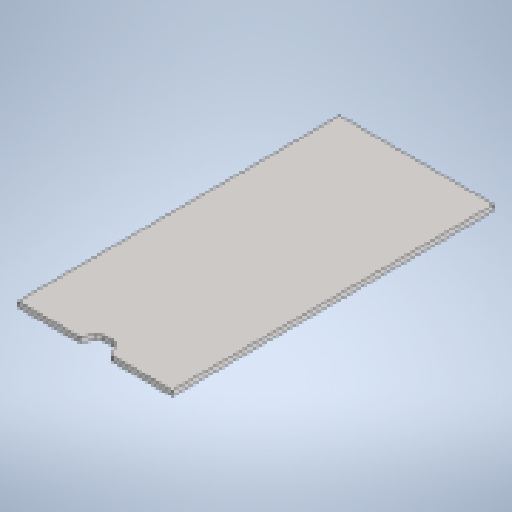
# Autodesk Inventor part: поперечная грань тела
Saved by Autodesk Inventor 2023.1 (Build 271208000, 208)
## iProperties
Created: 2024-11-21
Part Number: поперечная грань тела
Material: Типовые
Document SubType Name: Modeling
Designer: DELL
Density: 1 g/cm^3
Appearance: По умолчанию
Author: DELL
Autodesk Inventor part; units mm, degrees
ref_plane "YZ Plane" through (0, 0, 0) normal (1, 0, 0) x (0, 1, 0)
ref_plane "XZ Plane" through (0, 0, 0) normal (0, 1, 0) x (-1, 0, 0)
ref_plane "XY Plane" through (0, 0, 0) normal (0, 0, 1) x (1, 0, 0)
sketch "Эскиз1" plane through (0, 0, 0) normal (0, 0, 1) x (1, 0, 0)
  line L0 (60, 2) -> (-60, 2)
  line L1 (-60, 2) -> (-60, -2)
  line L2 (-60, -2) -> (60, -2)
  line L3 (60, -2) -> (60, 2)
  line L4 (60, 2) -> (-60, -2) construction
  line L5 (-60, 2) -> (60, -2) construction
  point P0 (0, 0)
  dimension "d0" = 120
  dimension "d1" = 4
  constraints: 12 end point, 2 midpoint, 2 parallel, 1 horizontal, 1 perpendicular
  measures "d0" distance of L2.end L1.end
  measures "d1" distance of L1.end L0.end
extrude "Выдавливание1" add sketch "Эскиз1" along normal blind 250
sketch "Эскиз2" plane through (-60, 2, 0) normal (0, 1, 0) x (1, 0, 0)
  line L0 (39.0177, -248.4604) -> (47.6438, -232.9811)
  line L1 (52.0114, -230.415) -> (65.6925, -230.415)
  line L2 (70.0601, -232.9811) -> (79.336, -249.6263)
  arc A0 (79.336, -249.6263) -> (79.5824, -250) centre (81.9565, -248.166) ccw
  arc A1 (36.3971, -250) -> (39.0177, -248.4604) centre (36.3971, -247) ccw
  arc A2 (70.0601, -232.9811) -> (65.6925, -230.415) centre (65.6925, -235.415) ccw
  arc A3 (52.0114, -230.415) -> (47.6438, -232.9811) centre (52.0114, -235.415) ccw
  line L3 (79.5824, -250) -> (36.3971, -250)
  line L4 (0, -250) -> (120, -250) projected
  line L5 (120, -250) -> (0, -250) projected
  point P0 (60, 0)
  point P1 (58.852, -247.058)
  point P2 (39.5541, -247.4978)
  point P3 (49.0738, -230.415)
  point P4 (68.6301, -230.415)
  point P5 (78.1498, -247.4978)
  point P6 (60, -250)
  point P7 (60, -250)
  dimension "d9" = 3
  dimension "d10" = 5
  dimension "d11" = 19.585
  constraints: 8 end point, 8 point on circle, 7 point on line, 7 tangent, 4 centre point, 2 equal radius, 1 horizontal, 1 midpoint, 8 other
  measures "d9" radius of A0
  measures "d10" radius of A2
  measures "d11" distance between parallel lines of L3 L1
extrude "Выдавливание2" cut sketch "Эскиз2" against normal blind 4
